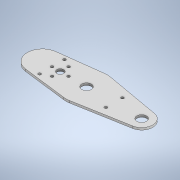
# Autodesk Inventor part: bottombeanv2
Saved by Autodesk Inventor 2020 (Build 240168000, 168)
## iProperties
Created: 2020-01-04
Part Number: bottombeanv2
Material: Generic
Document SubType Name: Modeling
Designer: xj82b
Density: 1 g/cm^3
Appearance: Default
Author: xj82b
Autodesk Inventor part; units mm, degrees
ref_plane "YZ Plane" through (0, 0, 0) normal (1, 0, 0) x (0, 1, 0)
ref_plane "XZ Plane" through (0, 0, 0) normal (0, 1, 0) x (-1, 0, 0)
ref_plane "XY Plane" through (0, 0, 0) normal (0, 0, 1) x (1, 0, 0)
sketch "Sketch1" plane through (0, 0, 0) normal (0, 1, 0) x (-1, 0, 0)
  line L0 (62.5322, -45.6018) -> (-188.8149, -45.6018) construction
  arc A0 (-158.4408, -29.8487) -> (-158.4408, -61.3549) centre (-155.6408, -45.6018) ccw
  arc A1 (-8.8908, -67.4293) -> (-8.8908, -23.7744) centre (-11.6408, -45.6018) ccw
  line L1 (-8.8908, -67.4293) -> (-71.8908, -75.3665)
  line L2 (-8.8908, -23.7744) -> (-71.8908, -15.8371)
  line L3 (-80.8908, -75.1389) -> (-158.4408, -61.3549)
  line L4 (-158.4408, -29.8487) -> (-80.8908, -16.0647)
  arc A2 (-80.8908, -75.1389) -> (-71.8908, -75.3665) centre (-75.6408, -45.6018) ccw
  arc A3 (-71.8908, -15.8371) -> (-80.8908, -16.0647) centre (-75.6408, -45.6018) ccw
  circle A4 centre (-155.6408, -45.6018) radius 7
  circle A5 centre (-75.6408, -45.6018) radius 7
  circle A6 centre (-37.5408, -45.6018) radius 12 construction
  circle A7 centre (-25.5408, -45.6018) radius 2
  circle A8 centre (-37.5408, -33.6018) radius 2
  circle A9 centre (-49.5408, -45.6018) radius 2
  circle A10 centre (-37.5408, -57.6018) radius 2
  circle A11 centre (-75.6408, -45.6018) radius 38.1 construction
  circle A12 centre (-155.6408, -45.6018) radius 38.1 construction
  circle A13 centre (-37.5408, -45.6018) radius 5
  circle A14 centre (-11.6408, -45.6018) radius 16 construction
  circle A15 centre (-25.5408, -63.6018) radius 2
  circle A16 centre (-25.5408, -27.6018) radius 2
  circle A17 centre (-115.6408, -57.6018) radius 2
  circle A18 centre (-115.6408, -33.6018) radius 2
  point P0 (0, 0)
  dimension "d9" = 24
  dimension "d16" = 76.2
  dimension "d0" = 32
  dimension "d1" = 44
  dimension "d3" = 80
  dimension "d4" = 64
  dimension "d5" = 14
  dimension "d6" = 14
  dimension "d7" = 30
  dimension "d8" = 30
  dimension "d10" = 4
  dimension "d13" = 360
  dimension "d15" = 12
  dimension "d17" = 76.2
  dimension "d18" = 10
  dimension "d19" = 32
  dimension "d20" = 4
  dimension "d21" = 4
  dimension "d22" = 4
  dimension "d23" = 4
  dimension "d24" = 40
  dimension "d25" = 40
  dimension "d26" = 12
  dimension "d27" = 12
  dimension "d30" = 36
  dimension "d31" = 18
  constraints: 17 centre point, 10 end point, 8 point on circle, 8 tangent, 6 coincident, 4 point on line, 2 horizontal alignment, 2 vertical alignment, 1 horizontal, 13 other
  measures "d0" diameter of A0
  measures "d1" diameter of A1
  measures "d3" distance of A2.centre A0.centre
  measures "d4" distance of A1.centre A2.centre
  measures "d5" diameter of A4
  measures "d6" diameter of A5
  measures "d7" radius of A2
  measures "d8" radius of A3
  measures "d10" diameter of A7
  measures "d15" distance from line of L0 A10.centre
  measures "d17" diameter of A12
  measures "d18" diameter of A13
  measures "d19" diameter of A14
  measures "d20" diameter of A15
  measures "d21" diameter of A16
  measures "d22" diameter of A17
  measures "d23" diameter of A18
  measures "d24" horizontal distance of A2.centre A17.centre
  measures "d25" horizontal distance of A2.centre A18.centre
  measures "d26" distance from line of L0 A17.centre
  measures "d27" distance from line of L0 A18.centre
  measures "d30" distance of A16.centre A15.centre
  measures "d31" distance from line of L0 A15.centre
extrude "Extrusion1" add sketch "Sketch1" along normal blind 3.175
body "Solid1"
